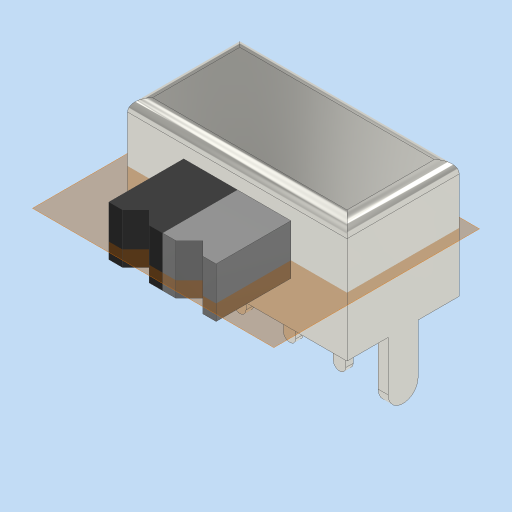
# Autodesk Inventor part: Power_switch
Saved by Autodesk Inventor 2024 (Build 280153000, 153)
## iProperties
Created: 2025-03-24
Part Number: Power_switch
Material: Generic
Document SubType Name: Modeling
Designer: XxPan
Density: 1 g/cm^3
Appearance: Default
Author: XxPan
Autodesk Inventor part; units mm, degrees
ref_plane "YZ Plane" through (0, 0, 0) normal (1, 0, 0) x (0, 1, 0)
ref_plane "XY Plane" through (0, 0, 0) normal (0, 0, 1) x (1, 0, 0)
sketch "Sketch1" plane through (0, 0, 0) normal (0, 0, 1) x (1, 0, 0)
  line L0 (-4.4, 2.375) -> (4.4, 2.375)
  line L1 (4.4, 2.375) -> (4.4, -2.375)
  line L2 (4.4, -2.375) -> (-4.4, -2.375)
  line L3 (-4.4, -2.375) -> (-4.4, 2.375)
  line L4 (-6.16, 0) -> (6.16, 0) construction
  line L5 (0, -3.325) -> (0, 3.325) construction
  point P0 (0, 0)
  dimension "d0" = 8.8
  dimension "d1" = 4.75
  constraints: 8 end point, 2 parallel, 1 horizontal, 1 perpendicular, 2 other
  measures "d0" distance of L0.start L0.end
  measures "d1" distance of L0.end L1.end
extrude "Extrusion1" add sketch "Sketch1" along normal mid plane 4.5
sketch "Sketch2" plane through (0, 0, 2.25) normal (0, 0, 1) x (1, 0, 0)
  line L0 (-2.15, 1.375) -> (2.15, 1.375)
  line L1 (2.15, 1.375) -> (2.15, -0.625)
  line L2 (2.15, -0.625) -> (-2.15, -0.625)
  line L3 (-2.15, -0.625) -> (-2.15, 1.375)
  line L4 (0, -3.325) -> (0, 3.325) construction
  line L5 (-6.16, 0) -> (6.16, 0) construction
  line L6 (4.4, 2.375) -> (-4.4, 2.375) projected
  point P0 (0, 0)
  dimension "d4" = 4.3
  dimension "d5" = 2
  dimension "d30" = 1
  constraints: 8 end point, 2 parallel, 1 horizontal, 1 perpendicular, 1 other
  measures "d4" distance of L1.end L2.end
  measures "d5" distance of L0.end L1.end
  measures "d30" distance between parallel lines of L6 L0
extrude "Extrusion2" add sketch "Sketch2" along normal blind 3
ref_plane "Work Plane1" through (0, -0.625, 2.25) normal (1, 0, 0) x (0, 0, -1)
split_face "Split1"
sketch "Sketch6" plane through (-2.15, 1.375, 2.25) normal (0, 1, 0) x (1, 0, 0)
  line L0 (2.15, -3) -> (0, -3) projected
  line L1 (0.5375, -3) -> (1.075, -2.4625)
  line L2 (1.075, -2.4625) -> (1.6125, -3)
  line L3 (0, -3) -> (2.15, -3) projected
  point P0 (2.15, 2.25)
  point P1 (1.075, -3)
  point P2 (1.075, -3)
  dimension "d24" = 2.15
  dimension "d25" = 0.5375
  dimension "d26" = 45
  constraints: 4 end point, 2 midpoint, 2 point on line, 1 perpendicular, 1 vertical alignment
  measures "d24" distance of L0.start L0.end
  measures "d25" distance of L1.start point (1.075, -3)
  measures "d26" angle of L0 L1
extrude "Extrusion4" cut sketch "Sketch6" against normal up to surface (2 mm away)
mirror "Mirror1" about plane through (0, -0.625, 2.25) normal (1, 0, 0) of "Extrusion4"
sketch "Sketch3" plane through (-4.4, -2.375, 2.25) normal (0, -1, 0) x (1, 0, 0)
  line L0 (0, -4.5) -> (0, 0) construction
  line L1 (0, -1.65) -> (0.4, -1.65)
  line L2 (0.4, -1.65) -> (0.4, -2.85)
  line L3 (0.4, -2.85) -> (0, -2.85)
  line L4 (0, -2.85) -> (0, -1.65)
  line L5 (8.8, -4.5) -> (8.8, 0) construction
  line L6 (8.8, -1.65) -> (8.4, -1.65)
  line L7 (8.4, -1.65) -> (8.4, -2.85)
  line L8 (8.4, -2.85) -> (8.8, -2.85)
  line L9 (8.8, -2.85) -> (8.8, -1.65)
  line L10 (4.15, -2.1) -> (4.65, -2.1)
  line L11 (4.65, -2.1) -> (4.65, -2.4)
  line L12 (4.65, -2.4) -> (4.15, -2.4)
  line L13 (4.15, -2.4) -> (4.15, -2.1)
  line L14 (2.15, -2.1) -> (2.65, -2.1)
  line L15 (2.65, -2.1) -> (2.65, -2.4)
  line L16 (2.65, -2.4) -> (2.15, -2.4)
  line L17 (2.15, -2.4) -> (2.15, -2.1)
  line L18 (6.15, -2.1) -> (6.65, -2.1)
  line L19 (6.65, -2.1) -> (6.65, -2.4)
  line L20 (6.65, -2.4) -> (6.15, -2.4)
  line L21 (6.15, -2.4) -> (6.15, -2.1)
  line L22 (-1.76, -2.25) -> (10.56, -2.25) construction
  line L23 (4.4, -6) -> (4.4, 4.5) construction
  point P0 (4.4, -2.25)
  dimension "d8" = 0.4
  dimension "d9" = 1.2
  dimension "d10" = 0.4
  dimension "d11" = 0.5
  dimension "d12" = 0.3
  dimension "d13" = 0.5
  dimension "d14" = 0.3
  dimension "d15" = 0.5
  dimension "d16" = 0.3
  dimension "d17" = 1.5
  constraints: 40 end point, 10 parallel, 5 horizontal, 5 perpendicular, 4 collinear, 2 point on line, 4 other
  measures "d8" distance of L2.end L3.end
  measures "d9" distance of L1.end L2.end
  measures "d10" distance of L8.end L7.end
  measures "d11" distance of L11.end L12.end
  measures "d12" distance of L10.end L11.end
  measures "d13" distance of L15.end L16.end
  measures "d14" distance of L14.end L15.end
  measures "d15" distance of L19.end L20.end
  measures "d16" distance of L18.end L19.end
  measures "d17" distance between parallel lines of L13 L15
extrude "Extrusion3" add sketch "Sketch3" along normal blind 2.6
fillet "Fillet1" radius 0.6 4 edges at (4.2, -4.975, 0.6) (4.2, -4.975, -0.6) (-4.2, -4.975, -0.6) (-4.2, -4.975, 0.6)
fillet "Fillet2" radius 0.25 6 edges at (2.25, -4.975, 0) (1.75, -4.975, 0) (0.25, -4.975, 0) (-0.25, -4.975, 0) (-1.75, -4.975, 0) (-2.25, -4.975, 0)
fillet "Fillet3" radius 0.5 4 edges at (4.4, 2.375, 0) (-4.4, 2.375, 0) (0, 2.375, 2.25) (0, 2.375, -2.25)
equation "\"d25\" = 0.25 * d24"
body "Solid1"
